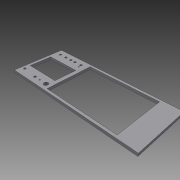
# Autodesk Inventor part: main_lcd_front_2
Saved by Autodesk Inventor 2014 (Build 180170000, 170)
## iProperties
Created: 2014-03-22
Part Number: main_lcd_front_2
Material: Generic
Document SubType Name: Modeling
Designer: buben
Density: 1 g/cm^3
Appearance: Default
Author: buben
Autodesk Inventor part; units mm, degrees
ref_plane "YZ Plane" through (0, 0, 0) normal (1, 0, 0) x (0, 1, 0)
ref_plane "XZ Plane" through (0, 0, 0) normal (0, 1, 0) x (-1, 0, 0)
ref_plane "XY Plane" through (0, 0, 0) normal (0, 0, 1) x (1, 0, 0)
sketch "Sketch1" plane through (0, 0, 0) normal (0, 1, 0) x (-1, 0, 0)
  line L0 (0, 0) -> (-300, 0)
  line L1 (-300, 0) -> (-300, -120)
  line L2 (-300, -120) -> (0, -120)
  line L3 (0, -120) -> (0, 0)
  line L4 (-96.5, -114) -> (-258.5, -114)
  line L5 (-258.5, -114) -> (-258.5, -6)
  line L6 (-258.5, -6) -> (-96.5, -6)
  line L7 (-96.5, -6) -> (-96.5, -114)
  circle A0 centre (-10, -17.5) radius 3
  circle A1 centre (-49, -14.1) radius 3
  circle A2 centre (-64, -14.1) radius 1.5
  circle A3 centre (-83, -14.1) radius 5.5
  circle A4 centre (-64, -14.1) radius 5.85 construction
  line L8 (-46, -17.1) -> (-52, -17.1) construction
  line L9 (-52, -17.1) -> (-52, -11.1) construction
  line L10 (-52, -11.1) -> (-46, -11.1) construction
  line L11 (-46, -11.1) -> (-46, -17.1) construction
  line L12 (-76.25, -20.1) -> (-89.75, -20.1) construction
  line L13 (-89.75, -20.1) -> (-89.75, -8.1) construction
  line L14 (-89.75, -8.1) -> (-76.25, -8.1) construction
  line L15 (-76.25, -8.1) -> (-76.25, -20.1) construction
  line L16 (-7.5, -84) -> (-86.5, -84)
  line L17 (-86.5, -84) -> (-86.5, -32)
  line L18 (-86.5, -32) -> (-7.5, -32)
  line L19 (-7.5, -32) -> (-7.5, -84)
  line L20 (-8, -83.5) -> (-86, -83.5) construction
  line L21 (-86, -83.5) -> (-86, -32.5) construction
  line L22 (-86, -32.5) -> (-8, -32.5) construction
  line L23 (-8, -32.5) -> (-8, -83.5) construction
  line L24 (-0.5, -93) -> (-93.5, -93) construction
  line L25 (-93.5, -93) -> (-93.5, -6) construction
  line L26 (-93.5, -6) -> (-0.5, -6) construction
  line L27 (-0.5, -6) -> (-0.5, -93) construction
  point P0 (-49, -17.1)
  point P1 (-52, -14.1)
  point P2 (-83, -20.1)
  point P3 (-89.75, -14.1)
  point P4 (-47, -83.5)
  point P5 (-47, -84)
  point P6 (-86, -58)
  point P7 (-86.5, -58)
  dimension "d0" = 300
  dimension "d1" = 6
  dimension "d4" = 3
  dimension "d5" = 11
  dimension "d6" = 6
  dimension "d7" = 19
  dimension "d8" = 15
  dimension "d9" = 11.7
  dimension "d10" = 6
  dimension "d11" = 13.5
  dimension "d12" = 12
  dimension "d15" = 162
  dimension "d16" = 108
  dimension "d18" = 6
  dimension "d19" = 6
  dimension "d20" = 79
  dimension "d21" = 52
  dimension "d22" = 78
  dimension "d23" = 51
  dimension "d24" = 18.4
  dimension "d25" = 7.5
  dimension "d27" = 87
  dimension "d28" = 9.5
  dimension "d29" = 10
  dimension "d30" = 0.5
  dimension "d33" = 6
  dimension "d34" = 15
  dimension "d35" = 9.5
  dimension "d36" = 10.5
  dimension "d37" = 93
  constraints: 56 end point, 14 parallel, 8 midpoint, 8 perpendicular, 7 horizontal, 5 centre point, 5 horizontal alignment, 3 vertical alignment, 1 coincident
  measures "d0" distance of L0.start L0.end
  measures "d1" diameter of A0
  measures "d4" diameter of A2
  measures "d5" diameter of A3
  measures "d6" diameter of A1
  measures "d7" distance of A3.centre A2.centre
  measures "d8" distance of A2.centre A1.centre
  measures "d9" diameter of A4
  measures "d10" distance of L9.end L10.end
  measures "d11" distance of L13.end L14.end
  measures "d12" distance of L12.end L13.end
  measures "d15" distance of L5.end L6.end
  measures "d16" distance of L6.end L4.start
  measures "d18" distance between parallel lines of L6 L0
  measures "d19" distance between parallel lines of L2 L4
  measures "d20" distance of L17.end L18.end
  measures "d21" distance of L18.end L16.start
  measures "d22" distance of L21.end L22.end
  measures "d23" distance of L22.end L20.start
  measures "d24" vertical distance of L21.end A3.centre
  measures "d25" distance between parallel lines of L23 L27
  measures "d27" distance of L26.end L24.start
  measures "d28" distance between parallel lines of L24 L20
  measures "d29" distance between parallel lines of L17 L7
  measures "d30" distance between parallel lines of L3 L27
  measures "d33" distance between parallel lines of L0 L26
  measures "d34" distance from line of L22 A0.centre
  measures "d35" distance from line of A0.centre L27
  measures "d36" distance from line of L25 A3.centre
  measures "d37" distance of L24.start L24.end
extrude "Extrusion1" add sketch "Sketch1" along normal blind 6.5
sketch "Sketch2" plane through (0, 6.5, 0) normal (0, 1, 0) x (1, 0, 0)
  line L0 (7.5, 84) -> (86.5, 84) projected
  circle A0 centre (14.518, 105.096) radius 3
  circle A1 centre (32.775, 105.096) radius 3
  circle A2 centre (60.989, 105.096) radius 3
  circle A3 centre (78.996, 105.096) radius 3
  circle A4 centre (48.582, 105.096) radius 3
  circle A5 centre (80.796, 97.596) radius 1.5
  line L1 (9, 110.1) -> (85, 110.1) construction
  line L2 (85, 110.1) -> (85, 94) construction
  line L3 (85, 94) -> (9, 94) construction
  line L4 (9, 94) -> (9, 110.1) construction
  point P0 (47, 84)
  point P1 (47, 94)
  dimension "d38" = 6
  dimension "d39" = 18.257
  dimension "d40" = 15.807
  dimension "d41" = 12.407
  dimension "d42" = 18.007
  dimension "d43" = 3
  dimension "d44" = 1.8
  dimension "d45" = 7.5
  dimension "d46" = 76
  dimension "d47" = 16.1
  dimension "d48" = 5.004
  dimension "d49" = 5.518
  dimension "d50" = 10
  constraints: 8 end point, 6 centre point, 4 equal radius, 4 horizontal alignment, 2 midpoint, 2 parallel, 1 horizontal, 1 perpendicular, 1 vertical alignment
  measures "d38" diameter of A0
  measures "d39" distance of A1.centre A0.centre
  measures "d40" distance of A4.centre A1.centre
  measures "d41" distance of A2.centre A4.centre
  measures "d42" distance of A3.centre A2.centre
  measures "d43" diameter of A5
  measures "d44" horizontal distance of A5.centre A3.centre
  measures "d45" vertical distance of A5.centre A3.centre
  measures "d46" distance of L2.end L3.end
  measures "d47" distance of L3.end L1.start
  measures "d48" distance from line of A0.centre L1
  measures "d49" distance from line of L4 A0.centre
  measures "d50" distance between parallel lines of L0 L3
extrude "Extrusion2" cut sketch "Sketch2" against normal through all
body "Solid1"
